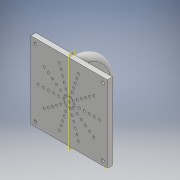
# Autodesk Inventor part: Top
Saved by Autodesk Inventor 2018 (Build 220112000, 112)
## iProperties
Created: 2018-04-10
Part Number: Top
Material: Generic
Document SubType Name: Modeling
Designer: a
Density: 1 g/cm^3
Appearance: Default
Author: a
## iProperties of the stored document Top_3DPrint.ipt
Created: 2018-04-10
Part Number: Top_3DPrint
Material: Generic
Document SubType Name: Modeling
Designer: a
Density: 1 g/cm^3
Appearance: Default
Author: a
Autodesk Inventor part; units mm, degrees
ref_plane "YZ Plane" through (0, 0, 0) normal (1, 0, 0) x (0, 1, 0)
ref_plane "XZ Plane" through (0, 0, 0) normal (0, 1, 0) x (-1, 0, 0)
ref_plane "XY Plane" through (0, 0, 0) normal (0, 0, 1) x (1, 0, 0)
sketch "Sketch1" plane through (0, 0, 0) normal (0, 1, 0) x (-1, 0, 0)
  line L0 (0, 0) -> (150, 0)
  line L1 (150, 0) -> (150, 150)
  line L2 (150, 150) -> (0, 150)
  line L3 (0, 150) -> (0, 0)
  dimension "d0" = 150
  dimension "d1" = 150
  constraints: 8 end point, 2 parallel, 1 horizontal, 1 perpendicular
  measures "d0" distance of L2.end L1.end
  measures "d1" distance of L1.end L0.end
extrude "Extrusion1" add sketch "Sketch1" along normal blind 10
sketch "Sketch2" plane through (0, 10, 0) normal (0, 1, 0) x (1, 0, 0)
  line L0 (-150, 0) -> (-150, -150) projected
  line L1 (0, -150) -> (0, 0) projected
  circle A0 centre (-75, -75) radius 70.3905
  circle A1 centre (-75, -75) radius 2
  dimension "d4" = 4
  constraints: 2 centre point, 1 coincident
  measures "d4" diameter of A1
extrude "Extrusion2" cut sketch "Sketch2" against normal blind 10 contours A1
pattern_linear "Rectangular Pattern1" count 7 spacing 10 along (1, 0, 0) count 7 spacing 10 along (-1, 0, 0) of "Extrusion2"
pattern_circular "Circular Pattern1" count 10 over 360 about axis through (-75, 10, 75) along (0, -1, 0) of "Extrusion2", "Rectangular Pattern1"
sketch "Sketch3" plane through (0, 10, 0) normal (0, 1, 0) x (1, 0, 0)
  line L0 (0, -150) -> (0, 0) projected
  line L1 (0, 0) -> (-8.8388, -8.8388)
  line L2 (0, 0) -> (12.5, 0) construction
  circle A0 centre (-8.8388, -8.8388) radius 2.82
  dimension "d16" = 12.5
  dimension "d17" = 135
  constraints: 4 end point, 1 centre point, 1 coincident, 1 equal length, 1 horizontal
  measures "d16" distance of L0.end L1.end
  measures "d17" angle of L1 L2
extrude "Extrusion3" cut sketch "Sketch3" against normal blind 10
pattern_linear "Rectangular Pattern2" count 2 spacing 132 along (0, 0, 1) count 2 spacing 132 along (-1, 0, 0) of "Extrusion3"
sketch "Sketch4" plane through (0, 10, 0) normal (0, 1, 0) x (1, 0, 0)
  line L0 (0, 0) -> (-150, 0) projected
  circle A0 centre (-75, -15.4654) radius 10.1579
  constraints: 1 centre point
sketch "Sketch5" plane through (0, 10, 0) normal (0, 1, 0) x (1, 0, 0)
  point P0 (0, 0)
sketch "Sketch6" plane through (0, 0, 0) normal (1, 0, 0) x (0, 1, 0)
  point P0 (0, 0)
ref_plane "Work Plane1" through (-75, 0, 150) normal (1, 0, 0) x (0, 0, -1)
sketch "Sketch7" plane through (-75, 0, 150) normal (1, 0, 0) x (0, 0, -1)
  arc A0 (134.5501, 9.9769) -> (14.3556, 10) centre (74.4532, 11.8101) ccw
  point P0 (150, 0)
  constraints: 2 point on circle, 1 centre point
sweep "Sweep1" add profiles "Sketch4" path "Sketch7"
body "Solid1"
